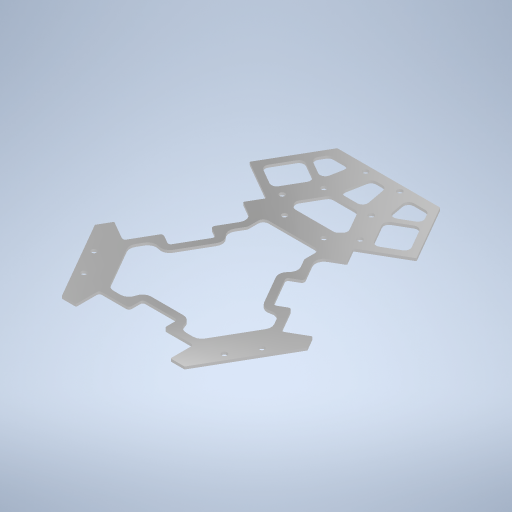
# Autodesk Inventor part: base_plate
Saved by Autodesk Inventor 2024.1 (Build 281209000, 209)
## iProperties
Created: 2025-02-03
Part Number: base_plate
Material: アルミニウム 6061
Document SubType Name: Sheet Metal
Designer: hibik
Density: 2.7 g/cm^3
Sheet Metal Rule: Default_mm
Appearance: アルミニウム - フラット
Author: hibik
Autodesk Inventor part; units mm, degrees
ref_plane "YZ Plane" through (0, 0, 0) normal (1, 0, 0) x (0, 1, 0)
ref_plane "XZ Plane" through (0, 0, 0) normal (0, 1, 0) x (-1, 0, 0)
ref_plane "XY Plane" through (0, 0, 0) normal (0, 0, 1) x (1, 0, 0)
sketch "スケッチ1" plane through (0, 0, 0) normal (0, 1, 0) x (-1, 0, 0)
  line L0 (75, 0) -> (105, -51.9615)
  line L1 (-75, 0) -> (-105, -51.9615)
  line L2 (0, -218.2384) -> (0, 36.3731)
  line L3 (147, 0) -> (-147, 0)
  line L4 (37.5, -27) -> (-37.5, -27)
  line L5 (105, -51.9615) -> (30, -181.8653)
  line L6 (30, -181.8653) -> (-30, -181.8653)
  line L7 (-30, -181.8653) -> (-105, -51.9615)
  line L8 (75, 0) -> (-75, 0)
  line L9 (-25.3673, -135.8894) -> (-62.8673, -70.9375)
  line L10 (25.3673, -135.8894) -> (62.8673, -70.9375)
  line L11 (-37.5, -27) -> (-27.5, -27)
  line L12 (-27.5, -27) -> (-27.5, -39)
  line L13 (-27.5, -39) -> (-37.5, -39)
  line L14 (-37.5, -39) -> (-37.5, -27)
  line L15 (37.5, -27) -> (27.5, -27)
  line L16 (27.5, -27) -> (27.5, -39)
  line L17 (27.5, -39) -> (37.5, -39)
  line L18 (37.5, -39) -> (37.5, -27)
  line L19 (0, -77.9423) -> (44.1173, -103.4134) construction
  line L20 (0, -77.9423) -> (-44.1173, -103.4134) construction
  line L21 (-44.1173, -103.4134) -> (-67.5, -116.9134) construction
  line L22 (-57.8673, -79.5977) -> (-47.475, -73.5977)
  line L23 (-52.475, -64.9375) -> (-62.8673, -70.9375)
  line L24 (-62.8673, -70.9375) -> (-57.8673, -79.5977)
  line L25 (-47.475, -73.5977) -> (-52.475, -64.9375)
  line L26 (-25.3673, -135.8894) -> (-30.3673, -127.2291)
  line L27 (-19.975, -121.2291) -> (-14.975, -129.8894)
  line L28 (-14.975, -129.8894) -> (-25.3673, -135.8894)
  line L29 (-30.3673, -127.2291) -> (-19.975, -121.2291)
  line L30 (30.3673, -127.2291) -> (19.975, -121.2291)
  line L31 (14.975, -129.8894) -> (25.3673, -135.8894)
  line L32 (25.3673, -135.8894) -> (30.3673, -127.2291)
  line L33 (19.975, -121.2291) -> (14.975, -129.8894)
  line L34 (62.8673, -70.9375) -> (57.8673, -79.5977)
  line L35 (47.475, -73.5977) -> (52.475, -64.9375)
  line L36 (52.475, -64.9375) -> (62.8673, -70.9375)
  line L37 (57.8673, -79.5977) -> (47.475, -73.5977)
  line L38 (62.8673, -70.9375) -> (37.5, -27)
  line L39 (-37.5, -27) -> (-62.8673, -70.9375)
  line L40 (-25.3673, -135.8894) -> (25.3673, -135.8894)
  line L41 (-25.3673, -135.8894) -> (-25.3673, -181.8653)
  line L42 (25.3673, -135.8894) -> (25.3673, -181.8653)
  line L43 (-25.3673, -135.8894) -> (-48.75, -149.3894)
  line L44 (25.3673, -135.8894) -> (48.75, -149.3894)
  point P0 (0, 0)
  point P1 (0, 0)
  point P2 (0, -27)
  dimension "d1" = 150
  dimension "d2" = 60
  dimension "d3" = 60
  dimension "d4" = 27
  dimension "d5" = 75
  dimension "d6" = 60
  dimension "d7" = 27
  dimension "d8" = 10
  dimension "d9" = 12
  dimension "d10" = 10
  dimension "d11" = 12
  dimension "d14" = 360
  measures "d1" distance of L1.start L0.start
  measures "d2" angle of L3 L0
  measures "d3" angle of L1 L3
  measures "d4" distance between parallel lines of L3 L4
  measures "d5" distance of L4.start L4.end
  measures "d6" distance of L5.end L6.end
  measures "d7" distance between parallel lines of L7 L9
  measures "d8" distance of L12.end L13.end
  measures "d9" distance of L11.end L12.end
  measures "d10" distance of L17.end L16.end
  measures "d11" distance of L16.end L15.end
extrude "プレート1" add sketch "スケッチ1" along normal blind 1.5 contours L5 L6 L42 L44 | L4 L16 L17 L18 L38 L36 L35 L37 L10 L30 L33 L31 L40 L2 | L2 L40 L28 L27 L29 L9 L22 L25 L23 L39 L14 L13 L12 L4 | L31 L33 L30 L10 | L42 L6 L2 L40 | L2 L6 L41 L40 | L4 L18 L17 L16 | L12 L13 L14 L4 | L9 L29 L27 L28 | L41 L6 L7 L43 | L37 L35 L36 L10 | L23 L25 L22 L9
sketch "スケッチ2" plane through (0, 0, 0) normal (0, -1, 0) x (1, 0, 0)
  line L0 (23.3798, -38.55) -> (-23.3798, -38.55) projected
  line L1 (8.2, -46.6) -> (-8.2, -46.6) projected
  arc A0 (-21.1, -27) -> (-23.3798, -38.55) centre (-21.1, -33) ccw projected
  line L2 (-27.5, -27) -> (-27.5, -39) projected
  line L3 (27.5, -39) -> (27.5, -27) projected
  line L4 (-27.5, -39) -> (-27.5, -40.55)
  line L5 (-27.5, -40.55) -> (-10.2, -40.55)
  line L6 (-10.2, -40.55) -> (-10.2, -48.6)
  line L7 (-10.2, -48.6) -> (10.2, -48.6)
  line L8 (10.2, -48.6) -> (10.2, -40.55)
  line L9 (10.2, -40.55) -> (27.5, -40.55)
  line L10 (27.5, -40.55) -> (27.5, -39)
  line L11 (-37.5, -27) -> (-27.5, -27) projected
  line L12 (-37.5, -27) -> (37.5, -27) projected
  line L13 (-20.3112, -101.4469) -> (-30.5112, -83.78)
  line L14 (-27.2827, -105.4719) -> (-20.3112, -101.4469)
  line L15 (-18.6327, -120.4541) -> (-27.2827, -105.4719)
  line L16 (-19.975, -121.2291) -> (-18.6327, -120.4541)
  line L17 (-37.4827, -87.805) -> (-46.1327, -72.8227)
  line L18 (-46.1327, -72.8227) -> (-47.475, -73.5977)
  line L19 (-30.5112, -83.78) -> (-37.4827, -87.805)
  line L20 (30.5112, -83.78) -> (20.3112, -101.4469)
  line L21 (37.4827, -87.805) -> (30.5112, -83.78)
  line L22 (46.1327, -72.8227) -> (37.4827, -87.805)
  line L23 (47.475, -73.5977) -> (46.1327, -72.8227)
  line L24 (27.2827, -105.4719) -> (18.6327, -120.4541)
  line L25 (18.6327, -120.4541) -> (19.975, -121.2291)
  line L26 (20.3112, -101.4469) -> (27.2827, -105.4719)
  line L27 (-47.475, -73.5977) -> (-57.8673, -79.5977)
  line L28 (-57.8673, -79.5977) -> (-30.3673, -127.2291)
  line L29 (-30.3673, -127.2291) -> (-19.975, -121.2291)
  line L30 (19.975, -121.2291) -> (30.3673, -127.2291)
  line L31 (30.3673, -127.2291) -> (57.8673, -79.5977)
  line L32 (57.8673, -79.5977) -> (47.475, -73.5977)
  point P0 (0, 0)
  point P1 (0, -77.9423)
  point P2 (-23.0432, -100.7148)
  point P3 (-33.5673, -121.6866)
  point P4 (-22.4248, -117.8859)
  point P5 (-25.3673, -135.8894)
  point P6 (-28.3712, -118.6866)
  point P7 (-31.2432, -86.512)
  point P8 (-45.8046, -77.3909)
  point P9 (-62.8673, -70.9375)
  point P10 (31.2432, -86.512)
  point P11 (54.6673, -85.1403)
  point P12 (45.8046, -77.3909)
  point P13 (62.8673, -70.9375)
  point P14 (49.4712, -82.1403)
  point P15 (23.0432, -100.7148)
  point P16 (22.4248, -117.8859)
  point P17 (25.3673, -135.8894)
  dimension "d17" = 2
  dimension "d18" = 2
  dimension "d19" = 2
  dimension "d20" = 2
  dimension "d26" = 360
  constraints: 54 end point, 9 perpendicular, 1 collinear, 1 horizontal, 1 vertical, 76 other
  measures "d17" distance between parallel lines of L0 L5
  measures "d18" distance from line of L1.end L6
  measures "d19" distance from line of L8 L1.start
  measures "d20" distance between parallel lines of L7 L1
extrude "切り取り1" cut sketch "スケッチ2" against normal blind 1.5
fillet "フィレット1" radius 1.5 16 edges at (-10.2, 0.75, -48.6) (-10.2, 0.75, -40.55) (-27.5, 0.75, -40.55) (10.2, 0.75, -48.6) (10.2, 0.75, -40.55) (27.5, 0.75, -40.55) (-30.5112, 0.75, -83.78) (-46.1327, 0.75, -72.8227) (-20.3112, 0.75, -101.4469) (-27.2827, 0.75, -105.4719) (-37.4827, 0.75, -87.805) (20.3112, 0.75, -101.4469) (27.2827, 0.75, -105.4719) (30.5112, 0.75, -83.78) (37.4827, 0.75, -87.805) (46.1327, 0.75, -72.8227)
sketch "スケッチ3" plane through (0, 0, 0) normal (0, -1, 0) x (1, 0, 0)
  circle A0 centre (40.9875, -45.0405) radius 1.6 projected
  circle A1 centre (48.9875, -58.8969) radius 1.6 projected
  circle A2 centre (-48.9875, -58.8969) radius 1.6 projected
  circle A3 centre (-40.9875, -45.0405) radius 1.6 projected
  point P0 (0, 0)
extrude "切り取り2" cut sketch "スケッチ3" against normal blind 1.5
sketch "スケッチ5" plane through (0, 1.5, 0) normal (0, 1, 0) x (1, 0, 0)
  line L0 (-19.975, 121.2291) -> (19.975, 121.2291) projected
  line L1 (47.475, 73.5977) -> (27.5, 39) projected
  line L2 (-47.475, 73.5977) -> (-27.5, 39) projected
  point P0 (0, 0)
sketch "スケッチ6" plane through (0, 1.5, 0) normal (0, 1, 0) x (1, 0, 0)
  line L0 (-26.0855, 44.55) -> (-41.9613, 72.0477)
  line L1 (-41.9613, 72.0477) -> (-36.0186, 82.3409)
  line L2 (-36.0186, 82.3409) -> (-29.0471, 78.3159)
  line L3 (-29.0471, 78.3159) -> (-14.8471, 102.911)
  line L4 (-14.8471, 102.911) -> (-21.8186, 106.936)
  line L5 (-21.8186, 106.936) -> (-15.8758, 117.2291)
  line L6 (-15.8758, 117.2291) -> (15.8758, 117.2291)
  line L7 (15.8758, 117.2291) -> (21.8186, 106.936)
  line L8 (21.8186, 106.936) -> (14.8471, 102.911)
  line L9 (14.8471, 102.911) -> (29.0471, 78.3159)
  line L10 (29.0471, 78.3159) -> (36.0186, 82.3409)
  line L11 (36.0186, 82.3409) -> (41.9613, 72.0477)
  line L12 (41.9613, 72.0477) -> (26.0855, 44.55)
  line L13 (26.0855, 44.55) -> (14.2, 44.55)
  line L14 (14.2, 44.55) -> (14.2, 52.6)
  line L15 (14.2, 52.6) -> (-14.2, 52.6)
  line L16 (-14.2, 52.6) -> (-14.2, 44.55)
  line L17 (-14.2, 44.55) -> (-26.0855, 44.55)
  line L18 (-47.475, 73.5977) -> (-27.5, 39) projected
  line L19 (-38.2327, 86.5059) -> (-45.3827, 74.1218) projected
  line L20 (-31.8102, 84.53) -> (-36.1836, 87.055) projected
  line L21 (-21.0612, 100.1479) -> (-29.7612, 85.079) projected
  line L22 (-25.9836, 104.7219) -> (-21.6102, 102.1969) projected
  line L23 (-18.6327, 120.4541) -> (-26.5327, 106.7709) projected
  line L24 (-19.975, 121.2291) -> (19.975, 121.2291) projected
  line L25 (47.475, 73.5977) -> (27.5, 39) projected
  line L26 (26.5327, 106.7709) -> (18.6327, 120.4541) projected
  line L27 (21.6102, 102.1969) -> (25.9836, 104.7219) projected
  line L28 (29.7612, 85.079) -> (21.0612, 100.1479) projected
  line L29 (36.1836, 87.055) -> (31.8102, 84.53) projected
  line L30 (45.3827, 74.1218) -> (38.2327, 86.5059) projected
  line L31 (11.7, 40.55) -> (26, 40.55) projected
  line L32 (10.2, 47.1) -> (10.2, 42.05) projected
  line L33 (-8.7, 48.6) -> (8.7, 48.6) projected
  line L34 (-10.2, 42.05) -> (-10.2, 47.1) projected
  line L35 (-26, 40.55) -> (-11.7, 40.55) projected
  line L36 (0, 48.6) -> (0, 121.2291)
  line L37 (-25.4112, 92.6134) -> (-31.0836, 95.8884) construction
  point P0 (0, 0)
  point P1 (-19.3827, 119.1551)
  point P2 (19.3827, 119.1551)
  dimension "d32" = 4
  dimension "d33" = 4
  dimension "d34" = 4
  dimension "d35" = 4
  dimension "d36" = 4
  dimension "d37" = 4
  dimension "d38" = 4
  dimension "d39" = 4
  dimension "d40" = 4
  constraints: 40 end point, 22 parallel, 3 midpoint, 3 perpendicular, 1 horizontal, 9 other
  measures "d32" distance between parallel lines of L19 L1
  measures "d33" distance between parallel lines of L18 L0
  measures "d34" distance between parallel lines of L21 L3
  measures "d35" distance from line of L20.start L2
  measures "d36" distance between parallel lines of L23 L5
  measures "d37" distance between parallel lines of L24 L6
  measures "d38" distance between parallel lines of L33 L15
  measures "d39" distance from line of L34.end L16
  measures "d40" distance between parallel lines of L35 L17
extrude "切り取り4" cut sketch "スケッチ6" against normal blind 1.5
fillet "フィレット2" radius 5 9 edges at (-14.2, 0.75, -44.55) (-26.0855, 0.75, -44.55) (-41.9613, 0.75, -72.0477) (-36.0186, 0.75, -82.3409) (-21.8186, 0.75, -106.936) (-15.8758, 0.75, -117.2291) (-14.2, 0.75, -52.6) (-29.0471, 0.75, -78.3159) (-14.8471, 0.75, -102.911)
mirror "ミラー1" about plane through (0, 0, 0) normal (1, 0, 0) of "フィレット2"
sketch "スケッチ7" plane through (0, 1.5, 0) normal (0, 1, 0) x (1, 0, 0)
  line L0 (16.5, 117.2291) -> (-16.5, 117.2291)
  line L1 (-16.5, 117.2291) -> (-16.5, 125.2291)
  line L2 (-16.5, 125.2291) -> (16.5, 125.2291)
  line L3 (16.5, 125.2291) -> (16.5, 117.2291)
  line L4 (-12.9891, 117.2291) -> (12.9891, 117.2291) projected
  line L5 (16.5, 117.2291) -> (16.5, 115.7891)
  arc A0 (17.3192, 114.7291) -> (12.9891, 117.2291) centre (12.9891, 112.2291) ccw projected
  line L6 (-16.5, 117.2291) -> (-16.5, 115.7891)
  arc A1 (-12.9891, 117.2291) -> (-17.3192, 114.7291) centre (-12.9891, 112.2291) ccw projected
  point P0 (0, 0)
  point P1 (0, 117.2291)
  dimension "d44" = 33
  dimension "d45" = 8
  constraints: 12 end point, 2 midpoint, 2 parallel, 2 point on circle, 2 vertical, 1 horizontal, 1 perpendicular
  measures "d44" distance of L1.end L2.end
  measures "d45" distance between parallel lines of L0 L2
extrude "切り取り5" cut sketch "スケッチ7" against normal blind 1.5
fillet "フィレット3" radius 3 4 edges at (-16.5, 0.75, -115.7891) (-16.5, 0.75, -125.2291) (16.5, 0.75, -125.2291) (16.5, 0.75, -115.7891)
fillet "フィレット4" radius 0.5 16 edges at (-48.75, 0.75, -149.3894) (-25.3673, 0.75, -135.8894) (-30.3673, 0.75, -127.2291) (-30, 0.75, -181.8653) (30, 0.75, -181.8653) (48.75, 0.75, -149.3894) (25.3673, 0.75, -135.8894) (30.3673, 0.75, -127.2291) (57.8673, 0.75, -79.5977) (62.8673, 0.75, -70.9375) (37.5, 0.75, -27) (27.5, 0.75, -27) (-27.5, 0.75, -27) (-37.5, 0.75, -27) (-62.8673, 0.75, -70.9375) (-57.8673, 0.75, -79.5977)
fillet "フィレット5" radius 5 2 edges at (18.6327, 0.75, -120.4541) (-18.6327, 0.75, -120.4541)
sketch "スケッチ8" plane through (0, 1.5, 0) normal (0, 1, 0) x (1, 0, 0)
  circle A0 centre (-40.9875, 45.0405) radius 1.6 projected
  circle A1 centre (48.9875, 58.8969) radius 1.6 projected
  circle A2 centre (40.9875, 45.0405) radius 1.6 projected
  circle A3 centre (-48.9875, 58.8969) radius 1.6 projected
  arc A4 (16.5, 116.8775) -> (17.0584, 115.1344) centre (19.5, 116.8775) ccw projected
  arc A5 (17.3192, 114.7291) -> (17.0584, 115.1344) centre (12.9891, 112.2291) ccw projected
  line L0 (17.3192, 114.7291) -> (19.3186, 111.2661) projected
  arc A6 (18.2848, 105.0066) -> (19.3186, 111.2661) centre (14.9884, 108.7661) ccw projected
  arc A7 (18.2848, 105.0066) -> (17.2511, 98.7471) centre (21.5812, 101.2471) ccw projected
  line L1 (17.2511, 98.7471) -> (26.643, 82.4797) projected
  arc A8 (26.643, 82.4797) -> (32.5808, 80.2452) centre (30.9732, 84.9797) ccw projected
  arc A9 (38.5186, 78.0107) -> (32.5808, 80.2452) centre (34.1884, 75.5107) ccw projected
  line L2 (38.5186, 78.0107) -> (40.5179, 74.5477) projected
  arc A10 (40.5179, 69.5477) -> (40.5179, 74.5477) centre (36.1878, 72.0477) ccw projected
  line L3 (40.5179, 69.5477) -> (27.5289, 47.05) projected
  arc A11 (23.1987, 44.55) -> (27.5289, 47.05) centre (23.1987, 49.55) ccw projected
  line L4 (23.1987, 44.55) -> (19.2, 44.55) projected
  arc A12 (14.296, 48.575) -> (19.2, 44.55) centre (19.2, 49.55) ccw projected
  arc A13 (14.296, 48.575) -> (9.392, 52.6) centre (9.392, 47.6) ccw projected
  line L5 (9.392, 52.6) -> (-9.392, 52.6) projected
  arc A14 (-9.392, 52.6) -> (-14.296, 48.575) centre (-9.392, 47.6) ccw projected
  arc A15 (-19.2, 44.55) -> (-14.296, 48.575) centre (-19.2, 49.55) ccw projected
  line L6 (-19.2, 44.55) -> (-23.1987, 44.55) projected
  arc A16 (-27.5289, 47.05) -> (-23.1987, 44.55) centre (-23.1987, 49.55) ccw projected
  line L7 (-27.5289, 47.05) -> (-40.5179, 69.5477) projected
  arc A17 (-40.5179, 74.5477) -> (-40.5179, 69.5477) centre (-36.1878, 72.0477) ccw projected
  line L8 (-40.5179, 74.5477) -> (-38.5186, 78.0107) projected
  arc A18 (-32.5808, 80.2452) -> (-38.5186, 78.0107) centre (-34.1884, 75.5107) ccw projected
  arc A19 (-32.5808, 80.2452) -> (-26.643, 82.4797) centre (-30.9732, 84.9797) ccw projected
  line L9 (-26.643, 82.4797) -> (-17.2511, 98.7471) projected
  arc A20 (-17.2511, 98.7471) -> (-18.2848, 105.0066) centre (-21.5812, 101.2471) ccw projected
  arc A21 (-19.3186, 111.2661) -> (-18.2848, 105.0066) centre (-14.9884, 108.7661) ccw projected
  line L10 (-19.3186, 111.2661) -> (-17.3192, 114.7291) projected
  arc A22 (-17.0584, 115.1344) -> (-17.3192, 114.7291) centre (-12.9891, 112.2291) ccw projected
  arc A23 (-17.0584, 115.1344) -> (-16.5, 116.8775) centre (-19.5, 116.8775) ccw projected
  line L11 (-16.5, 116.8775) -> (-16.5, 122.2291) projected
  arc A24 (-13.5, 125.2291) -> (-16.5, 122.2291) centre (-13.5, 122.2291) ccw projected
  line L12 (-13.5, 125.2291) -> (13.5, 125.2291) projected
  arc A25 (16.5, 122.2291) -> (13.5, 125.2291) centre (13.5, 122.2291) ccw projected
  line L13 (16.5, 122.2291) -> (16.5, 116.8775) projected
  arc A26 (-57.4343, 79.3477) -> (-58.1173, 79.1647) centre (-57.6843, 78.9147) ccw projected
  line L14 (-62.723, 71.1875) -> (-58.1173, 79.1647) projected
  arc A27 (-62.723, 71.1875) -> (-62.723, 70.6875) centre (-62.29, 70.9375) ccw projected
  line L15 (-37.6443, 27.25) -> (-62.723, 70.6875) projected
  arc A28 (-37.6443, 27.25) -> (-37.2113, 27) centre (-37.2113, 27.5) ccw projected
  line L16 (-28, 27) -> (-37.2113, 27) projected
  arc A29 (-28, 27) -> (-27.5, 27.5) centre (-28, 27.5) ccw projected
  line L17 (-27.5, 27.5) -> (-27.5, 39.05) projected
  arc A30 (-26, 40.55) -> (-27.5, 39.05) centre (-26, 39.05) ccw projected
  line L18 (-26, 40.55) -> (-11.7, 40.55) projected
  arc A31 (-11.7, 40.55) -> (-10.2, 42.05) centre (-11.7, 42.05) ccw projected
  line L19 (-10.2, 42.05) -> (-10.2, 47.1) projected
  arc A32 (-8.7, 48.6) -> (-10.2, 47.1) centre (-8.7, 47.1) ccw projected
  line L20 (-8.7, 48.6) -> (8.7, 48.6) projected
  arc A33 (10.2, 47.1) -> (8.7, 48.6) centre (8.7, 47.1) ccw projected
  line L21 (10.2, 47.1) -> (10.2, 42.05) projected
  arc A34 (10.2, 42.05) -> (11.7, 40.55) centre (11.7, 42.05) ccw projected
  line L22 (11.7, 40.55) -> (26, 40.55) projected
  arc A35 (27.5, 39.05) -> (26, 40.55) centre (26, 39.05) ccw projected
  line L23 (27.5, 39.05) -> (27.5, 27.5) projected
  arc A36 (27.5, 27.5) -> (28, 27) centre (28, 27.5) ccw projected
  line L24 (37.2113, 27) -> (28, 27) projected
  arc A37 (37.2113, 27) -> (37.6443, 27.25) centre (37.2113, 27.5) ccw projected
  line L25 (62.723, 70.6875) -> (37.6443, 27.25) projected
  arc A38 (62.723, 70.6875) -> (62.723, 71.1875) centre (62.29, 70.9375) ccw projected
  line L26 (58.1173, 79.1647) -> (62.723, 71.1875) projected
  arc A39 (58.1173, 79.1647) -> (57.4343, 79.3477) centre (57.6843, 78.9147) ccw projected
  line L27 (57.4343, 79.3477) -> (47.4317, 73.5727) projected
  arc A40 (45.3827, 74.1218) -> (47.4317, 73.5727) centre (46.6817, 74.8718) ccw projected
  line L28 (45.3827, 74.1218) -> (38.2327, 86.5059) projected
  arc A41 (38.2327, 86.5059) -> (36.1836, 87.055) centre (36.9336, 85.7559) ccw projected
  line L29 (36.1836, 87.055) -> (31.8102, 84.53) projected
  arc A42 (29.7612, 85.079) -> (31.8102, 84.53) centre (31.0602, 85.829) ccw projected
  line L30 (29.7612, 85.079) -> (21.0612, 100.1479) projected
  arc A43 (21.6102, 102.1969) -> (21.0612, 100.1479) centre (22.3602, 100.8979) ccw projected
  line L31 (21.6102, 102.1969) -> (25.9836, 104.7219) projected
  arc A44 (25.9836, 104.7219) -> (26.5327, 106.7709) centre (25.2336, 106.0209) ccw projected
  line L32 (26.5327, 106.7709) -> (21.1327, 116.124) projected
  arc A45 (22.9628, 122.9541) -> (21.1327, 116.124) centre (25.4628, 118.624) ccw projected
  line L33 (22.9628, 122.9541) -> (29.9343, 126.9791) projected
  arc A46 (29.9343, 126.9791) -> (30.1173, 127.6621) centre (29.6843, 127.4121) ccw projected
  line L34 (25.6173, 135.4564) -> (30.1173, 127.6621) projected
  arc A47 (25.8003, 136.1394) -> (25.6173, 135.4564) centre (26.0503, 135.7064) ccw projected
  line L35 (48.317, 149.1394) -> (25.8003, 136.1394) projected
  arc A48 (48.317, 149.1394) -> (48.5, 149.8224) centre (48.067, 149.5724) ccw projected
  line L36 (30.1443, 181.6153) -> (48.5, 149.8224) projected
  arc A49 (30.1443, 181.6153) -> (29.7113, 181.8653) centre (29.7113, 181.3653) ccw projected
  line L37 (-29.7113, 181.8653) -> (29.7113, 181.8653) projected
  arc A50 (-29.7113, 181.8653) -> (-30.1443, 181.6153) centre (-29.7113, 181.3653) ccw projected
  line L38 (-48.5, 149.8224) -> (-30.1443, 181.6153) projected
  arc A51 (-48.5, 149.8224) -> (-48.317, 149.1394) centre (-48.067, 149.5724) ccw projected
  line L39 (-25.8003, 136.1394) -> (-48.317, 149.1394) projected
  arc A52 (-25.6173, 135.4564) -> (-25.8003, 136.1394) centre (-26.0503, 135.7064) ccw projected
  line L40 (-30.1173, 127.6621) -> (-25.6173, 135.4564) projected
  arc A53 (-30.1173, 127.6621) -> (-29.9343, 126.9791) centre (-29.6843, 127.4121) ccw projected
  line L41 (-29.9343, 126.9791) -> (-22.9628, 122.9541) projected
  arc A54 (-21.1327, 116.124) -> (-22.9628, 122.9541) centre (-25.4628, 118.624) ccw projected
  line L42 (-21.1327, 116.124) -> (-26.5327, 106.7709) projected
  arc A55 (-26.5327, 106.7709) -> (-25.9836, 104.7219) centre (-25.2336, 106.0209) ccw projected
  line L43 (-25.9836, 104.7219) -> (-21.6102, 102.1969) projected
  arc A56 (-21.0612, 100.1479) -> (-21.6102, 102.1969) centre (-22.3602, 100.8979) ccw projected
  line L44 (-21.0612, 100.1479) -> (-29.7612, 85.079) projected
  arc A57 (-31.8102, 84.53) -> (-29.7612, 85.079) centre (-31.0602, 85.829) ccw projected
  line L45 (-31.8102, 84.53) -> (-36.1836, 87.055) projected
  arc A58 (-36.1836, 87.055) -> (-38.2327, 86.5059) centre (-36.9336, 85.7559) ccw projected
  line L46 (-38.2327, 86.5059) -> (-45.3827, 74.1218) projected
  arc A59 (-47.4317, 73.5727) -> (-45.3827, 74.1218) centre (-46.6817, 74.8718) ccw projected
  line L47 (-47.4317, 73.5727) -> (-57.4343, 79.3477) projected
  line L48 (-62.0013, 72.4375) -> (-35.7679, 27)
  line L49 (35.7679, 27) -> (62.0013, 72.4375)
  line L50 (62.723, 70.6875) -> (37.6443, 27.25) projected
  line L51 (-37.6443, 27.25) -> (-62.723, 70.6875) projected
  line L52 (0, 218.308) -> (0, -36.3847) projected
  point P0 (0, 0)
  dimension "d51" = 1.5
  constraints: 4 end point, 4 point on line, 2 parallel, 1 other
  measures "d51" distance between parallel lines of L50 L49
extrude "切り取り6" cut sketch "スケッチ8" against normal blind 1.5 contours L16 A28 L15 A27 L14 L48 | L49 L26 A38 L25 A37 L24
sketch "スケッチ9" plane through (0, 0, 0) normal (0, -1, 0) x (1, 0, 0)
  circle A0 centre (11.5, -132.5985) radius 1.6 projected
  circle A1 centre (-11.5, -132.5985) radius 1.6 projected
  point P0 (0, 0)
extrude "切り取り7" cut sketch "スケッチ9" against normal blind 1.5
sketch "スケッチ19" plane through (0, 0, 0) normal (0, -1, 0) x (1, 0, 0)
  circle A0 centre (-10, -178.3653) radius 1.6
  circle A1 centre (-13.8342, -157.8653) radius 1.6
  circle A2 centre (-22.7342, -142.4501) radius 1.6
  line L0 (-13.8342, -157.8653) -> (-22.7342, -142.4501) construction
  line L1 (-30.1443, -181.6153) -> (-48.5, -149.8224) projected
  line L2 (-22.7342, -142.4501) -> (-25.213, -143.8812) construction
  line L3 (29.7113, -181.8653) -> (-29.7113, -181.8653) projected
  point P0 (0, 0)
  point P1 (0, -181.8653)
  dimension "d56" = 26
  dimension "d57" = 17.8
  dimension "d58" = 3.2
  dimension "d59" = 24
  dimension "d60" = 3.5
  dimension "d61" = 10
  constraints: 4 end point, 3 centre point, 2 equal radius, 1 coincident, 1 midpoint, 1 parallel, 1 perpendicular
  measures "d56" distance between parallel lines of L1 L0
  measures "d57" distance from line of L0.start L2
  measures "d58" diameter of A0
  measures "d59" distance from line of L3 L0.start
  measures "d60" distance from line of L3 A0.centre
  measures "d61" horizontal distance of point (0, -181.865) A0.centre
extrude "切り取り8" cut sketch "スケッチ19" against normal blind 1.5
mirror "ミラー2" about plane through (0, 0, 0) normal (1, 0, 0) of "切り取り8"
sketch "スケッチ20" plane through (0, 0, 0) normal (0, -1, 0) x (1, 0, 0)
  line L0 (15.9165, -142.2587) -> (12.2562, -138.5985)
  line L1 (12.2562, -138.5985) -> (-12.2562, -138.5985)
  line L2 (-12.2562, -138.5985) -> (-15.9165, -142.2587)
  line L3 (-15.9165, -142.2587) -> (-8.0607, -155.8653)
  line L4 (-8.0607, -155.8653) -> (8.0607, -155.8653)
  line L5 (8.0607, -155.8653) -> (15.9165, -142.2587)
  line L6 (4.27, -176.3653) -> (7.3561, -159.8653)
  line L7 (7.3561, -159.8653) -> (-7.3561, -159.8653)
  line L8 (-7.3561, -159.8653) -> (-4.27, -176.3653)
  line L9 (-4.27, -176.3653) -> (4.27, -176.3653)
  line L10 (28.5566, -176.3653) -> (16.4781, -176.3653)
  line L11 (16.4781, -176.3653) -> (19.5433, -159.9769)
  line L12 (19.5433, -159.9769) -> (29.4295, -142.8535)
  line L13 (29.4295, -142.8535) -> (43.2859, -150.8535)
  line L14 (43.2859, -150.8535) -> (28.5566, -176.3653)
  line L15 (-16.4781, -176.3653) -> (-28.5566, -176.3653)
  line L16 (-28.5566, -176.3653) -> (-43.2859, -150.8535)
  line L17 (-43.2859, -150.8535) -> (-29.4295, -142.8535)
  line L18 (-29.4295, -142.8535) -> (-19.5433, -159.9769)
  line L19 (-19.5433, -159.9769) -> (-16.4781, -176.3653)
  circle A0 centre (10, -178.3653) radius 1.6 projected
  circle A1 centre (13.8342, -157.8653) radius 1.6 projected
  circle A2 centre (22.7342, -142.4501) radius 1.6 projected
  circle A3 centre (-22.7342, -142.4501) radius 1.6 projected
  circle A4 centre (-13.8342, -157.8653) radius 1.6 projected
  circle A5 centre (-10, -178.3653) radius 1.6 projected
  line L20 (22.7342, -142.4501) -> (13.8342, -157.8653) construction
  line L21 (13.8342, -157.8653) -> (10, -178.3653) construction
  line L22 (-10, -178.3653) -> (-13.8342, -157.8653) construction
  line L23 (-13.8342, -157.8653) -> (-22.7342, -142.4501) construction
  line L24 (0, -218.2384) -> (0, 36.3731) projected
  circle A6 centre (11.5, -132.5985) radius 1.6 projected
  circle A7 centre (-11.5, -132.5985) radius 1.6 projected
  line L25 (11.5, -132.5985) -> (-11.5, -132.5985) construction
  line L26 (-30.1443, -181.6153) -> (-48.5, -149.8224) projected
  line L27 (-48.317, -149.1394) -> (-25.8003, -136.1394) projected
  line L28 (29.7113, -181.8653) -> (-29.7113, -181.8653) projected
  line L29 (32.6497, -169.2759) -> (34.1497, -166.6778)
  line L30 (34.1497, -166.6778) -> (20.2933, -158.6778)
  line L31 (20.2933, -158.6778) -> (18.7933, -161.2759)
  line L32 (18.7933, -161.2759) -> (32.6497, -169.2759)
  line L33 (-32.6497, -169.2759) -> (-34.1497, -166.6778)
  line L34 (-34.1497, -166.6778) -> (-20.2933, -158.6778)
  line L35 (-20.2933, -158.6778) -> (-18.7933, -161.2759)
  line L36 (-18.7933, -161.2759) -> (-32.6497, -169.2759)
  point P0 (0, 0)
  point P1 (19.2509, -161.5401)
  point P2 (-19.2509, -161.5401)
  dimension "d64" = 6
  dimension "d65" = 6
  dimension "d66" = 5
  dimension "d67" = 2
  dimension "d68" = 2
  dimension "d69" = 2
  dimension "d70" = 6
  dimension "d71" = 6
  dimension "d72" = 6
  dimension "d73" = 4
  dimension "d74" = 4
  dimension "d75" = 3
  constraints: 66 end point, 15 parallel, 5 point on line, 4 perpendicular, 3 horizontal, 2 midpoint, 10 other
  measures "d64" distance between parallel lines of L20 L5
  measures "d65" distance between parallel lines of L25 L1
  measures "d66" distance from line of L0.end L5
  measures "d67" distance from line of L22.end L4
  measures "d68" distance from line of L7 L22.end
  measures "d69" distance from line of L22.start L9
  measures "d70" distance between parallel lines of L22 L8
  measures "d71" distance between parallel lines of L22 L19
  measures "d72" distance between parallel lines of L23 L18
  measures "d73" distance between parallel lines of L26 L16
  measures "d74" distance between parallel lines of L27 L17
  measures "d75" distance between parallel lines of L34 L36
extrude "押し出し1" cut sketch "スケッチ20" against normal through all contours L5 L4 L24 L1 L0 | L24 L4 L3 L2 L1 | L9 L24 L7 L6 | L9 L8 L7 L24 | L10 L11 L32 L14 | L30 L12 L13 L14 | L15 L16 L36 L19 | L16 L17 L18 L34
fillet "フィレット6" radius 3 13 edges at (34.1497, 0.75, -166.6778) (20.2933, 0.75, -158.6778) (29.4295, 0.75, -142.8535) (43.2859, 0.75, -150.8535) (32.6497, 0.75, -169.2759) (28.5566, 0.75, -176.3653) (16.4781, 0.75, -176.3653) (19.2509, 0.75, -161.5401) (15.9165, 0.75, -142.2587) (8.0607, 0.75, -155.8653) (12.2562, 0.75, -138.5985) (7.3561, 0.75, -159.8653) (4.27, 0.75, -176.3653)
mirror "ミラー3" about plane through (0, 0, 0) normal (1, 0, 0) of "フィレット6"
equation "\"d3\" = d2"
equation "\"d7\" = d4"
equation "\"d19\" = d18"
equation "\"d21\" = Thickness"
equation "\"d28\" = Thickness"
equation "\"d33\" = d32"
equation "\"d34\" = d32"
equation "\"d35\" = d32"
equation "\"d36\" = d32"
equation "\"d37\" = d32"
equation "\"d38\" = d32"
equation "\"d39\" = d32"
equation "\"d40\" = d32"
equation "\"d41\" = Thickness"
equation "\"d46\" = Thickness"
equation "\"d52\" = Thickness"
equation "\"d54\" = Thickness"
equation "\"d62\" = Thickness"
equation "\"d65\" = d64"
equation "\"d68\" = d67"
equation "\"d70\" = d64"
equation "\"d71\" = d70"
equation "\"d72\" = d71"
equation "\"d74\" = d73"
equation "\"d16\" = Thickness"
equation "\"BendRadius\" = Thickness"
equation "\"BendReliefWidth\" = Thickness"
equation "\"BendReliefDepth\" = 0.5 * Thickness"
equation "\"CornerReliefSize\" = 4 * Thickness"
equation "\"MinimumRemnant\" = 2 * Thickness"
equation "\"TransitionRadius\" = BendRadius"
equation "\"JacobiRadiusSize\" = BendRadius"
equation "\"GapSize\" = Thickness"
equation "\"Thickness\" = 1.5"
